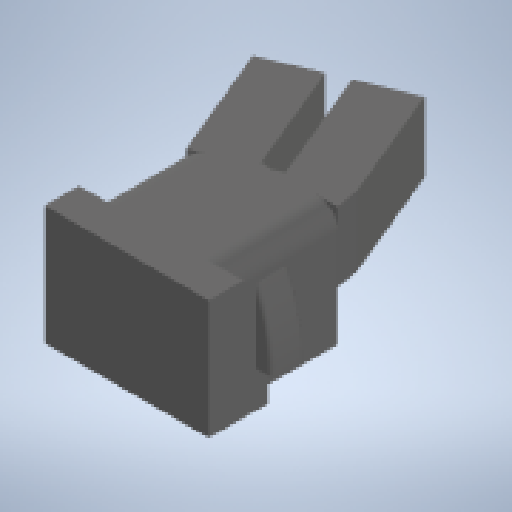
# Autodesk Inventor part: connector_male_bend_left
Saved by Autodesk Inventor 2026.1 (Build 301233020, 233B)
## iProperties
Created: 2025-09-28
Part Number: connector_male_bend_left
Material: 一般
Document SubType Name: Modeling
Designer: hibik
Density: 1 g/cm^3
Appearance: 既定
Author: hibik
Autodesk Inventor part; units mm, degrees
ref_plane "XZ Plane" through (0, 0, 0) normal (0, 1, 0) x (-1, 0, 0)
ref_plane "XY Plane" through (0, 0, 0) normal (0, 0, 1) x (1, 0, 0)
sketch "スケッチ1" plane through (0, 0, 0) normal (0, 1, 0) x (-1, 0, 0)
  line L0 (10, -0.3) -> (0, -0.3)
  line L1 (0, -0.3) -> (0, -5)
  line L2 (0, -5) -> (10, -5)
  line L3 (10, -5) -> (10, -0.3)
  line L4 (8.5, -5) -> (0, -5)
  line L5 (0, -5) -> (0, -18)
  line L6 (0, -18) -> (8.5, -18)
  line L7 (8.5, -18) -> (8.5, -5)
  line L8 (10, -18) -> (0, -18)
  line L9 (0, -18) -> (0, -22.7)
  line L10 (0, -22.7) -> (10, -22.7)
  line L11 (10, -22.7) -> (10, -18)
  point P0 (0, 0)
  dimension "d0" = 10
  dimension "d2" = 1.5
  dimension "d3" = 13
  dimension "d34" = 5
  dimension "d35" = 0.3
  constraints: 24 end point, 6 parallel, 5 collinear, 3 horizontal, 3 perpendicular, 2 point on line, 1 coincident
  measures "d0" distance of L0.start L0.end
  measures "d2" distance between parallel lines of L3 L7
  measures "d3" distance of L6.end L4.start
  measures "d34" distance from line of point (0, 0) L2
  measures "d35" distance from line of point (0, 0) L0
extrude "押し出し1" add sketch "スケッチ1" along normal blind 15
sketch "スケッチ3" plane through (-10, 0, -18) normal (0, 0, 1) x (1, 0, 0)
  line L0 (0, 0) -> (1.5, 0) projected
  line L1 (1.5, 0) -> (1.5, 15) projected
  line L2 (0, 15) -> (1.5, 15) projected
  line L3 (0, 0) -> (0, 15) projected
  line L4 (0, 0) -> (10, 0) projected
  line L5 (10, 0) -> (10, 15) projected
  line L6 (0, 15) -> (10, 15) projected
  line L7 (0, 0) -> (0, 15) projected
  circle A0 centre (4.5, 12) radius 3
  circle A1 centre (4.5, 12) radius 2.5
  line L8 (2, 12) -> (2, 0)
  line L9 (4.5, 14.5) -> (10, 14.5)
  point P0 (1.5, 15)
  point P1 (1.5, 0)
  dimension "d6" = 6
  dimension "d7" = 0.5
  constraints: 4 end point, 4 tangent, 2 centre point, 2 perpendicular, 2 point on circle, 2 point on line, 1 coincident
  measures "d6" diameter of A0
  measures "d7" radial gap between concentric circles of A0 A1
extrude "押し出し2" cut sketch "スケッチ3" along normal up to surface (13 mm away) contours L1 A0 L8 L4 | L1 L6 A0 | A0 L9 A1 L8 | L6 L5 L9 A0 picked at (5.4334, 14.5914)
sketch "スケッチ4" plane through (0, 15, 0) normal (0, 1, 0) x (1, 0, 0)
  line L0 (0, 5) -> (-10, 5) projected
  line L1 (-10, 5) -> (-10, 0.3) projected
  line L2 (-10, 0.3) -> (0, 0.3) projected
  line L3 (0, 0.3) -> (0, 5) projected
  point P0 (0, 0)
extrude "押し出し3" cut sketch "スケッチ4" against normal up to surface (0.5 mm away)
sketch "スケッチ5" plane through (-8, 0, -18) normal (-1, 0, 0) x (0, 0, 1)
  line L0 (13, 0) -> (18, 0) projected
  line L1 (13, 0) -> (3, 0)
  line L2 (3, 0) -> (3, 15)
  line L3 (3, 15) -> (13, 15)
  line L4 (13, 15) -> (13, 0)
  line L5 (6, 12) -> (10, 12)
  line L6 (10, 12) -> (10, 2)
  line L7 (10, 2) -> (6, 2)
  line L8 (6, 2) -> (6, 12)
  line L9 (13, 0) -> (0, 0) projected
  point P0 (6.5, 0)
  point P1 (8, 12)
  point P2 (8, 15)
  dimension "d12" = 10
  dimension "d13" = 3
  dimension "d14" = 2
  dimension "d15" = 4
  dimension "d21" = 15
  constraints: 16 end point, 4 parallel, 3 midpoint, 2 horizontal, 2 perpendicular, 1 vertical alignment
  measures "d12" distance of L2.end L3.end
  measures "d13" distance between parallel lines of L3 L5
  measures "d14" distance from line of point (6.5, 0) L7
  measures "d15" distance of L6.end L7.end
  measures "d21" distance of L1.end L2.end
extrude "押し出し4" add sketch "スケッチ5" along normal blind 2 contours L5 L6 L7 L8
sketch "スケッチ6" plane through (-8, 2, -8) normal (0, 0, 1) x (1, 0, 0)
  line L0 (0, 10) -> (0, 0) projected
  line L1 (0, 10) -> (-2, 10) projected
  line L2 (-2, 0) -> (-2, 10) projected
  line L3 (0, 0) -> (-2, 0) projected
  line L4 (0, 0) -> (0, 10) projected
  arc A0 (0, 9.5) -> (-2, 0.5) centre (19.25, 0.5) ccw
  line L5 (-2, 0.5) -> (0, 0.5)
  point P0 (8, -2)
  point P1 (0, 0.5)
  dimension "d22" = 0.5
  dimension "d23" = 0.5
  constraints: 3 point on line, 2 end point, 2 point on circle, 1 centre point, 1 perpendicular, 1 tangent
  measures "d22" distance from line of L1 A0.start
  measures "d23" distance from line of L3 L5.start
extrude "押し出し5" cut sketch "スケッチ6" against normal up to surface (4 mm away) contours L0 A0 L2 L1 | L0 L3 L2 L5
fillet "フィレット1" radius 0.5 2 edges at (-9.494, 7.1098, -12) (-9.494, 7.1098, -8)
mirror "ミラー1" about plane through (0, 0, -0.3) normal (1, 0, 0)
sketch "スケッチ7" plane through (-5.5, 14.5, -5) normal (0, 0, -1) x (-1, 0, 0)
  line L0 (4.5, 0) -> (0, 0) projected
  arc A0 (2.5, -2.5) -> (0, 0) centre (0, -2.5) ccw projected
  line L1 (2.5, -14.5) -> (2.5, -2.5) projected
  line L2 (4.5, -14.5) -> (2.5, -14.5) projected
  line L3 (4.5, -14.5) -> (4.5, 0) projected
  line L4 (-15.5, 0) -> (-11, 0) projected
  line L5 (-15.5, -14.5) -> (-15.5, 0) projected
  line L6 (-15.5, -14.5) -> (-13.5, -14.5) projected
  line L7 (-13.5, -14.5) -> (-13.5, -2.5) projected
  arc A1 (-11, 0) -> (-13.5, -2.5) centre (-11, -2.5) ccw projected
  point P0 (-5.5, -14.5)
extrude "押し出し6" cut sketch "スケッチ7" against normal blind 0.5
sketch "スケッチ13" plane through (-10, 14.5, -0.3) normal (0, 1, 0) x (1, 0, 0)
  arc A0 (21.586, 79.673) -> (5.1529, 40) centre (157.8276, 0) ccw projected
  arc A1 (46.2266, 111.6009) -> (0, 0) centre (157.8276, 0) ccw projected
  line L0 (0, 22.4) -> (0, 32.4) projected
  line L1 (0, 22.4) -> (0, 22.4) projected
  line L2 (0, 17.7) -> (0, 22.4) projected
  line L3 (0, 17.7) -> (2, 17.7) projected
  line L4 (0, 32.4) -> (20, 32.4) projected
  point P0 (10, -0.3)
  point P1 (0.9956, 17.7)
  point P2 (3.3615, 32.4)
extrude "押し出し14" cut sketch "スケッチ13" along normal through all both and the other way through all
mirror "ミラー2" about plane through (0, 0, 0) normal (1, 0, 0) of "押し出し14"
sketch "スケッチ14" plane through (0, 0, 0) normal (0, -1, 0) x (1, 0, 0)
  line L0 (1.5, -6) -> (-1.5, -6)
  line L1 (-1.5, -6) -> (-1.5, -16)
  line L2 (-1.5, -16) -> (1.5, -16)
  line L3 (1.5, -16) -> (1.5, -6)
  line L4 (5, -9.5) -> (-5, -9.5)
  line L5 (-5, -9.5) -> (-5, -12.5)
  line L6 (-5, -12.5) -> (5, -12.5)
  line L7 (5, -12.5) -> (5, -9.5)
  point P0 (0, 0)
  point P1 (5, -11)
  point P2 (1.5, -11)
  point P3 (0, -6)
  point P4 (0, -9.5)
  point P5 (1.5, -9.5)
  point P6 (-1.5, -9.5)
  point P7 (-1.5, -12.5)
  point P8 (1.5, -12.5)
  dimension "d65" = 10
  dimension "d66" = 3
  dimension "d70" = 6
  constraints: 16 end point, 4 midpoint, 4 parallel, 4 perpendicular, 2 horizontal, 2 vertical alignment, 1 horizontal alignment
  measures "d65" distance of L4.start L4.end
  measures "d66" distance of L6.end L4.start
  measures "d70" distance from line of point (0, 0) L0
extrude "押し出し15" add sketch "スケッチ14" along normal blind 5
sketch "スケッチ15" plane through (0, 0, 0) normal (0, -1, 0) x (1, 0, 0)
  arc A0 (-9.0044, -18) -> (-8.4023, -22.7) centre (147.8276, -0.3) ccw projected
  line L0 (-9.0044, -18) -> (9.0044, -18)
  line L1 (9.0044, -18) -> (9.0044, -22.7)
  line L2 (9.0044, -22.7) -> (-9.0044, -22.7)
  line L3 (-9.0044, -22.7) -> (-9.0044, -18)
  point P0 (0, 0)
  point P1 (8.4023, -22.7)
  constraints: 8 end point, 2 parallel, 1 horizontal, 1 perpendicular, 1 point on line
extrude "押し出し16" cut sketch "スケッチ15" against normal through all
ref_plane "作業平面1" through (0, 14.5, -18) normal (-0.3826834, 0, -0.9238795) x (0, -1, 0)
sketch "スケッチ19" plane through (0, 14.5, -18) normal (-0.3826834, 0, -0.9238795) x (0, -1, 0)
  line L0 (14.5, 8) -> (0, 8)
  line L1 (0, 8) -> (0, -8)
  line L2 (0, -8) -> (14.5, -8)
  line L3 (14.5, -8) -> (14.5, 8)
  line L4 (-3.9, 0) -> (23.4, 0) projected
  line L5 (14.5, 7.391) -> (14.5, -7.391) projected
  line L6 (0, 5.0813) -> (0, -5.0813) projected
  line L7 (0, 1.25) -> (14.5, 1.25)
  line L8 (14.5, 1.25) -> (14.5, -1.25)
  line L9 (14.5, -1.25) -> (0, -1.25)
  line L10 (0, -1.25) -> (0, 1.25)
  point P0 (14.5, 6.8883)
  point P1 (14.5, 0)
  point P2 (0, 0)
  point P3 (0, 0)
  point P4 (0, -1.25)
  point P5 (0, 1.25)
  dimension "d89" = 16
  dimension "d90" = 2.5
  constraints: 16 end point, 6 midpoint, 4 parallel, 3 point on line, 2 horizontal, 2 perpendicular
  measures "d89" distance of L2.end L0.start
  measures "d90" distance between parallel lines of L9 L7
extrude "押し出し20" add sketch "スケッチ19" along normal blind 15 contours L3 L7 L1 L0 | L3 L2 L1 L9
sketch "スケッチ21" plane through (1.1548, 14.5, -18.4784) normal (0, 1, 0) x (0.9238795, 0, -0.3826834)
  line L0 (0, 0) -> (6.75, 0) projected
  line L1 (-2.5, 0.5178) -> (3.8313, -2.1048) projected
  line L2 (3.8313, -2.1048) -> (6.141, -3.0615) projected
  line L3 (6.75, 0) -> (6.141, -3.0615)
  line L4 (0, 0) -> (-1.25, 0)
  point P0 (-8.1383, -16.6298)
  constraints: 4 end point, 1 horizontal, 1 point on line
extrude "押し出し22" add sketch "スケッチ21" against normal up to surface (14.5 mm away)
sketch "スケッチ22" plane through (-5.7403, 14.5, -31.8582) normal (-0.3826834, 0, -0.9238795) x (-0.9238795, 0, 0.3826834)
  line L0 (12.5573, -14.5) -> (8, -14.5) projected
  line L1 (-8, 0) -> (-8, -14.5) projected
  line L2 (8, -14.5) -> (-8, -14.5)
  line L3 (-8, -14.5) -> (-8, -8.5)
  line L4 (-8, -8.5) -> (8, -8.5)
  line L5 (8, -8.5) -> (8, -14.5)
  point P0 (6.8883, -14.5)
  point P1 (-8, -14.5)
  dimension "d97" = 6
  constraints: 8 end point, 2 parallel, 1 horizontal, 1 perpendicular, 1 point on line
  measures "d97" distance of L4.end L0.end
extrude "押し出し23" cut sketch "スケッチ22" against normal up to surface surface through (-9.0044, 0, -18) normal (0, 0, 1)
equation "\"d22\" = d23"
